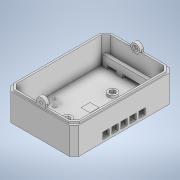
# Autodesk Inventor part: Casing-v2
Saved by Autodesk Inventor 2020 (Build 240168000, 168)
## iProperties
Created: 2020-11-24
Part Number: Casing-v2
Material: Generic
Document SubType Name: Modeling
Designer: Leon
Density: 1 g/cm^3
Appearance: Default
Author: Leon
Autodesk Inventor part; units mm, degrees
ref_plane "YZ Plane" through (0, 0, 0) normal (1, 0, 0) x (0, 1, 0)
ref_plane "XZ Plane" through (0, 0, 0) normal (0, 1, 0) x (-1, 0, 0)
ref_plane "XY Plane" through (0, 0, 0) normal (0, 0, 1) x (1, 0, 0)
sketch "Sketch1" plane through (0, 0, 0) normal (0, 1, 0) x (-1, 0, 0)
  line L0 (-37.5, -55) -> (37.5, -55)
  line L1 (37.5, -55) -> (37.5, 55)
  line L2 (37.5, 55) -> (-37.5, 55)
  line L3 (-37.5, 55) -> (-37.5, -55)
  line L4 (-37.5, -55) -> (37.5, 55) construction
  line L5 (37.5, -55) -> (-37.5, 55) construction
  point P0 (0, 0)
  dimension "d0" = 110
  dimension "d1" = 75
  constraints: 12 end point, 2 midpoint, 2 parallel, 1 horizontal, 1 perpendicular
  measures "d0" distance of L0.end L1.end
  measures "d1" distance of L0.start L0.end
extrude "Extrusion1" add sketch "Sketch1" along normal blind 30
shell "Shell1" thickness 3 removed faces 1 at (12.5, 30, 18.3333)
chamfer "Chamfer1" distance 5 angle 45 8 edges at (37.5, 15, 55) (-37.5, 15, 55) (-34.5, 16.5, 52) (-34.5, 16.5, -52) (-37.5, 15, -55) (37.5, 15, -55) (34.5, 16.5, -52) (34.5, 16.5, 52)
sketch "Sketch2" plane through (-34.5, 3, -52) normal (0, 1, 0) x (1, 0, 0)
  circle A0 centre (14, -70.5) radius 1.1 projected
  circle A1 centre (62, -79.5) radius 1.1 projected
  circle A2 centre (14, -70.5) radius 2
  circle A3 centre (62, -79.5) radius 2
  line L0 (2.5, -6.0253) -> (66.5, -6.0253)
  line L1 (66.5, -2.0253) -> (2.5, -2.0253)
  line L2 (2.5, -2.0253) -> (2.5, -6.0253)
  line L3 (66.5, -5.0253) -> (66.5, -89.5)
  line L4 (66.5, -6.0253) -> (66.5, -2.0253)
  point P0 (34.5, -52)
  point P1 (66.5, -4.0253)
  dimension "d5" = 4
  dimension "d6" = 4
  dimension "d34" = 4
  dimension "d157" = 64
  dimension "d158" = 1
  constraints: 10 end point, 3 vertical, 2 centre point, 2 coincident, 1 collinear, 1 horizontal, 1 midpoint, 1 parallel, 2 other
  measures "d5" diameter of A2
  measures "d6" diameter of A3
  measures "d34" distance between parallel lines of L1 L0
  measures "d157" distance of L0.end L0.start
  measures "d158" distance of L3.start point (66.5, -4.025)
ref_plane "Work Plane2" through (-32, 8, -42.5) normal (0, -1, 0) x (1, 0, 0)
extrude "Extrusion5" add sketch "Sketch2" along normal blind 7 contours A0 | A1 | A2 | A3 | L2 L1 L4 L3 L0
sketch "Sketch8" plane through (32, 3, -49.9747) normal (0, 0, -1) x (-1, 0, 0)
  line L0 (63.5253, 0) -> (0.4747, 0) projected
  line L1 (63.5253, 0) -> (0.4747, 0) projected
  line L2 (5, 0) -> (15, 0)
  line L3 (15, 0) -> (15, 4)
  line L4 (15, 4) -> (5, 4)
  line L5 (5, 4) -> (5, 0)
  line L6 (0, 0) -> (64, 0) projected
  line L7 (22, 0) -> (42, 0)
  line L8 (42, 0) -> (42, 4)
  line L9 (42, 4) -> (22, 4)
  line L10 (22, 4) -> (22, 0)
  line L11 (49, 0) -> (59, 0)
  line L12 (59, 0) -> (59, 4)
  line L13 (59, 4) -> (49, 4)
  line L14 (49, 4) -> (49, 0)
  line L15 (0.4747, 7) -> (63.5253, 7) projected
  line L16 (0.4747, 0) -> (0.4747, 7) projected
  line L17 (63.5253, 7) -> (63.5253, 0) projected
  point P0 (32, -3)
  point P1 (32, 4)
  point P2 (32, 7)
  dimension "d50" = 10
  dimension "d51" = 20
  dimension "d52" = 4
  dimension "d55" = 10
  constraints: 24 end point, 6 parallel, 5 point on line, 3 horizontal, 3 perpendicular, 2 horizontal alignment, 1 midpoint, 1 vertical alignment
  measures "d50" distance of L3.end L4.end
  measures "d51" distance of L8.end L9.end
  measures "d52" distance between parallel lines of L0 L4
  measures "d55" distance of L12.end L13.end
extrude "Extrusion7" cut sketch "Sketch8" against normal up to surface (4 mm away) contours L0 L14 L13 L12 | L0 L10 L9 L8 | L5 L4 L3 L0
sketch "Sketch10" plane through (0, 30, 0) normal (0, 1, 0) x (1, 0, 0)
  line L0 (-29.5, 52) -> (29.5, 52) projected
  line L1 (34.5, 47) -> (34.5, -47) projected
  line L2 (29.5, -52) -> (-29.5, -52) projected
  line L3 (-34.5, -47) -> (-34.5, 47) projected
  line L4 (-37.5, 50) -> (-37.5, -50) projected
  line L5 (-32.5, -55) -> (32.5, -55) projected
  line L6 (37.5, -50) -> (37.5, 50) projected
  line L7 (32.5, 55) -> (-32.5, 55) projected
  line L8 (32.5, 55) -> (37.5, 50) projected
  line L9 (-37.5, 50) -> (-32.5, 55) projected
  line L10 (-32.5, -55) -> (-37.5, -50) projected
  line L11 (37.5, -50) -> (32.5, -55) projected
  line L12 (-29.5, 52) -> (-34.5, 47) projected
  line L13 (34.5, 47) -> (29.5, 52) projected
  line L14 (29.5, -52) -> (34.5, -47) projected
  line L15 (-34.5, -47) -> (-29.5, -52) projected
  line L16 (-36.5, 47.8284) -> (-36.5, -47.8284)
  line L17 (-36.5, -47.8284) -> (-30.3284, -54)
  line L18 (-30.3284, -54) -> (30.3284, -54)
  line L19 (30.3284, -54) -> (36.5, -47.8284)
  line L20 (36.5, -47.8284) -> (36.5, 47.8284)
  line L21 (36.5, 47.8284) -> (30.3284, 54)
  line L22 (30.3284, 54) -> (-30.3284, 54)
  line L23 (-30.3284, 54) -> (-36.5, 47.8284)
  dimension "d126" = 2
  constraints: 16 end point, 7 other
  measures "d126" distance between parallel lines of L3 L16
extrude "Extrusion8" add sketch "Sketch10" along normal blind 2 contours L23 L22 L21 L20 L19 L18 L17 L16
sketch "Sketch15" plane through (37.5, 0, 55) normal (1, 0, 0) x (0, 0, -1)
  line L0 (5, 0) -> (105, 0) projected
  line L1 (5, 30) -> (105, 30) projected
  circle A0 centre (65, 6.5) radius 3.5 construction
  circle A1 centre (55, 6.5) radius 3.5 construction
  circle A2 centre (75, 6.5) radius 3.5 construction
  circle A3 centre (35, 6.5) radius 3.5 construction
  circle A4 centre (45, 6.5) radius 3.5 construction
  line L2 (31.5, 3) -> (38.5, 3)
  line L3 (38.5, 3) -> (38.5, 10)
  line L4 (38.5, 10) -> (31.5, 10)
  line L5 (31.5, 10) -> (31.5, 3)
  line L6 (31.5, 3) -> (38.5, 10) construction
  line L7 (38.5, 3) -> (31.5, 10) construction
  line L8 (41.5, 3) -> (48.5, 3)
  line L9 (48.5, 3) -> (48.5, 10)
  line L10 (48.5, 10) -> (41.5, 10)
  line L11 (41.5, 10) -> (41.5, 3)
  line L12 (41.5, 3) -> (48.5, 10) construction
  line L13 (48.5, 3) -> (41.5, 10) construction
  line L14 (51.5, 3) -> (58.5, 3)
  line L15 (58.5, 3) -> (58.5, 10)
  line L16 (58.5, 10) -> (51.5, 10)
  line L17 (51.5, 10) -> (51.5, 3)
  line L18 (51.5, 3) -> (58.5, 10) construction
  line L19 (58.5, 3) -> (51.5, 10) construction
  line L20 (61.5, 3) -> (68.5, 3)
  line L21 (68.5, 3) -> (68.5, 10)
  line L22 (68.5, 10) -> (61.5, 10)
  line L23 (61.5, 10) -> (61.5, 3)
  line L24 (61.5, 3) -> (68.5, 10) construction
  line L25 (68.5, 3) -> (61.5, 10) construction
  line L26 (71.5, 3) -> (78.5, 3)
  line L27 (78.5, 3) -> (78.5, 10)
  line L28 (78.5, 10) -> (71.5, 10)
  line L29 (71.5, 10) -> (71.5, 3)
  line L30 (71.5, 3) -> (78.5, 10) construction
  line L31 (78.5, 3) -> (71.5, 10) construction
  line L32 (105, 30) -> (105, 0) projected
  line L33 (5, 0) -> (5, 30) projected
  point P0 (55, 0)
  point P1 (55, 0)
  dimension "d71" = 7
  dimension "d72" = 7
  dimension "d73" = 7
  dimension "d77" = 6.5
  dimension "d90" = 7
  dimension "d91" = 7
  dimension "d92" = 10
  dimension "d94" = 10
  dimension "d95" = 10
  dimension "d96" = 10
  constraints: 60 end point, 11 midpoint, 10 parallel, 9 tangent, 5 centre point, 5 horizontal, 5 perpendicular, 4 horizontal alignment, 1 point on line, 1 vertical alignment
  measures "d71" diameter of A2
  measures "d72" diameter of A0
  measures "d73" diameter of A1
  measures "d77" distance from line of L0 A2.centre
  measures "d90" diameter of A4
  measures "d91" diameter of A3
  measures "d92" distance of A4.centre A3.centre
  measures "d94" distance of A1.centre A4.centre
  measures "d95" distance of A0.centre A1.centre
  measures "d96" distance of A0.centre A2.centre
extrude "Extrusion12" cut sketch "Sketch15" against normal up to surface (3 mm away) contours L5 L4 L3 L2 | L11 L10 L9 L8 | L17 L16 L15 L14 | L23 L22 L21 L20 | L29 L28 L27 L26
sketch "Sketch16" plane through (-34.5, 10, -52) normal (0, 1, 0) x (1, 0, 0)
  line L0 (2.5, -6.0253) -> (66.5, -6.0253) projected
  line L1 (66.0253, -2.0253) -> (2.9747, -2.0253) projected
  line L2 (2.5, -2.5) -> (2.5, -6.0253) projected
  line L3 (66.5, -4.2627) -> (2.5, -4.2627)
  line L4 (66.0253, -2.0253) -> (66.5, -2.5) projected
  line L5 (2.5, -2.5) -> (2.9747, -2.0253) projected
  line L6 (66.5, -6.0253) -> (66.5, -2.5) projected
  point P0 (34.5, -52)
  constraints: 2 end point, 1 midpoint
extrude "Extrusion13" add sketch "Sketch16" along normal blind 5
sketch "Sketch17" plane through (-20.5, 10, 18.5) normal (0, 1, 0) x (1, 0, 0)
  circle A0 centre (0, 0) radius 2 construction
  circle A1 centre (48, -9) radius 2 construction
  point P0 (20.5, 18.5)
hole "Hole3" at (-20.5, 10, 18.5) at (27.5, 10, 27.5) direction (0, -1, 0) diameter 1.9 depth 5
sketch "Sketch18" plane through (-34.5, 3, 52) normal (0, 1, 0) x (1, 0, 0)
  circle A0 centre (34.5, 27) radius 5
  line L0 (32.9123, 29.75) -> (36.0877, 29.75)
  line L1 (36.0877, 29.75) -> (37.6754, 27)
  line L2 (37.6754, 27) -> (36.0877, 24.25)
  line L3 (36.0877, 24.25) -> (32.9123, 24.25)
  line L4 (32.9123, 24.25) -> (31.3246, 27)
  line L5 (31.3246, 27) -> (32.9123, 29.75)
  line L6 (-3, 107) -> (-3, -3) projected
  line L7 (-3, -3) -> (72, -3) projected
  line L8 (72, -3) -> (72, 107) projected
  point P0 (34.5, 52)
  dimension "d97" = 5.5
  dimension "d98" = 10
  dimension "d114" = 25
  constraints: 12 end point, 1 centre point, 1 coincident, 1 horizontal, 1 vertical alignment, 13 other
  measures "d97" distance between parallel lines of L0 L3
  measures "d98" diameter of A0
  measures "d114" distance of point (34.5, 52) A0.centre
extrude "Extrusion14" add sketch "Sketch18" along normal blind 2.5
hole "Hole4" at (0, 3, 25) direction (0, -1, 0) diameter 3 depth 5
mirror "Mirror2" about plane through (0, 0, 0) normal (0, 0, 1) of "Extrusion14", "Hole4"
sketch "Sketch22" plane through (-29.5, 3, -52) normal (0, 0, 1) x (1, 0, 0)
  line L0 (59, 29) -> (59, 0) projected
  line L1 (0, 29) -> (59, 29) projected
  line L2 (0, 0) -> (0, 29) projected
  line L3 (59, 0) -> (0, 0) projected
  line L4 (32.6754, 31.75) -> (31.0877, 29)
  line L5 (31.0877, 29) -> (27.9123, 29)
  line L6 (27.9123, 29) -> (26.3246, 31.75)
  line L7 (26.3246, 31.75) -> (27.9123, 34.5)
  line L8 (27.9123, 34.5) -> (31.0877, 34.5)
  line L9 (31.0877, 34.5) -> (32.6754, 31.75)
  circle A0 centre (29.5, 31.75) radius 5
  line L10 (0, 29) -> (59, 29) projected
  line L11 (24.5, 31.75) -> (24.5, 29)
  line L12 (34.5, 31.75) -> (34.5, 29)
  line L13 (24.5, 29) -> (34.5, 29)
  line L14 (34.5, 29) -> (34.5, 24)
  line L15 (34.5, 24) -> (24.5, 24)
  line L16 (24.5, 24) -> (24.5, 29)
  point P0 (29.5, -3)
  point P1 (29.5, 29)
  point P2 (33.6758, 29)
  point P3 (25.3242, 29)
  dimension "d141" = 5.5
  dimension "d142" = 10
  dimension "d145" = 5
  constraints: 24 end point, 3 perpendicular, 2 collinear, 2 horizontal, 2 parallel, 2 point on circle, 2 point on line, 2 tangent, 1 centre point, 1 coincident, 1 midpoint, 1 vertical alignment, 13 other
  measures "d141" distance between parallel lines of L5 L8
  measures "d142" diameter of A0
  measures "d145" distance of L15.end L11.end
extrude "Extrusion19" add sketch "Sketch22" against normal blind 2 contours L14 L15 L16 L1 A0 | L1 A0 L12 | A0 L1 | L1 L4 L9 L8 L7 L6 A0 | L1 L6 L7 L8 L9 L4 | L1 L11 A0
extrude "Extrusion20" add sketch "Sketch22" along normal blind 2 contours A0 L1 | L1 L4 L9 L8 L7 L6 A0
hole "Hole6" at (0, 34.75, -52) direction (0, 0, -1) diameter 3 depth 5
mirror "Mirror3" about plane through (0, 0, 0) normal (0, 0, 1) of "Extrusion19", "Extrusion20", "Hole6"
sketch "Sketch23" plane through (-29.5, 3, -52) normal (0, 1, 0) x (1, 0, 0)
  line L0 (34.5, -57) -> (24.5, -57)
  line L1 (24.5, -57) -> (24.5, -47)
  line L2 (24.5, -47) -> (34.5, -47)
  line L3 (34.5, -47) -> (34.5, -57)
  line L4 (34.5, -57) -> (24.5, -47) construction
  line L5 (24.5, -57) -> (34.5, -47) construction
  point P0 (29.5, -52)
  dimension "d155" = 10
  dimension "d156" = 10
  constraints: 12 end point, 2 midpoint, 2 parallel, 1 horizontal, 1 perpendicular
  measures "d155" distance of L1.end L2.end
  measures "d156" distance of L0.end L1.end
split_face "Split1"
equation "\"d55\" = d50"
equation "\"d72\" = d71"
equation "\"d73\" = d71"
equation "\"d90\" = d73"
equation "\"d91\" = d73"
equation "\"d94\" = d75"
equation "\"d95\" = d94"
equation "\"d96\" = d95"
equation "\"d75\" = 10"
body "Solid1"
